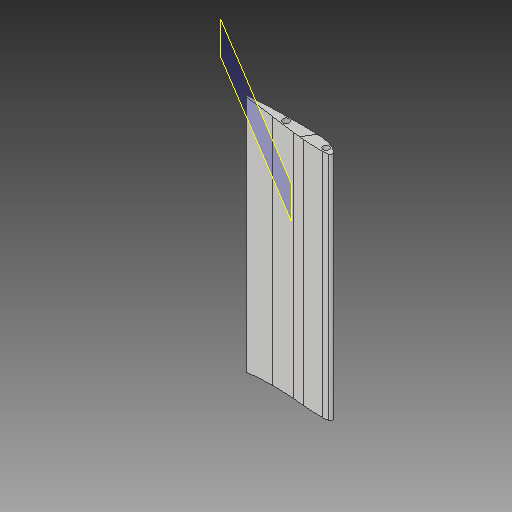
# Autodesk Inventor part: newsubflap_top
Saved by Autodesk Inventor 2018.3 (Build 223284000, 284)
## iProperties
Created: 2018-06-11
Part Number: newsubflap_top
Material: 一般
Document SubType Name: Modeling
Designer: ku_sk
Density: 1 g/cm^3
Appearance: 既定
Author: ku_sk
Autodesk Inventor part; units mm, degrees
ref_plane "YZ Plane" through (0, 0, 0) normal (1, 0, 0) x (0, 1, 0)
ref_plane "XZ Plane" through (0, 0, 0) normal (0, 1, 0) x (-1, 0, 0)
ref_plane "XY Plane" through (0, 0, 0) normal (0, 0, 1) x (1, 0, 0)
sketch "スケッチ1" plane through (0, 0, 0) normal (0, 1, 0) x (-1, 0, 0)
  circle A0 centre (56.6667, -3.3333) radius 2 projected
  circle A1 centre (6.6667, -1.3333) radius 2 projected
  arc A2 (27.618, -9.313) -> (80.2911, 0.2239) centre (24.5838, 157.671) ccw projected
  arc A3 (20.5062, -9.2317) -> (27.618, -9.313) centre (25.435, 110.8283) ccw projected
  arc A4 (7.5483, -6.9284) -> (20.5062, -9.2317) centre (22.5133, 39.66) ccw projected
  arc A5 (0.14, -3.2897) -> (7.5483, -6.9284) centre (16.2383, 20.125) ccw projected
  arc A6 (-1.8521, -1.3552) -> (0.14, -3.2897) centre (4.8333, 3.5367) ccw projected
  arc A7 (-0.4054, 2.2589) -> (-1.8521, -1.3552) centre (0, 0) ccw projected
  arc A8 (5.081, 2.7563) -> (-0.4054, 2.2589) centre (5.1833, -28.88) ccw projected
  arc A9 (23.6457, 1.9287) -> (5.081, 2.7563) centre (5.71, -191.7767) ccw projected
  arc A10 (23.6457, 1.9287) -> (35.0642, 0.89) centre (351.2983, 3540.5833) ccw projected
  arc A11 (35.0642, 0.89) -> (56.4197, -0.0064) centre (55.24, 226.7233) ccw projected
  arc A12 (56.4197, -0.0064) -> (79.9865, 1.514) centre (55.3817, 199.4967) ccw projected
  arc A13 (80.2911, 0.2239) -> (79.9865, 1.514) centre (80.0687, 0.8524) ccw projected
extrude "押し出し1" add sketch "スケッチ1" along normal mid plane 250 contours A0 | A1 | A3 A4 A5 A6 A7 A8 A9 A10 A11 A12 A13 A2
sketch "スケッチ2" plane through (0, -125, 0) normal (0, -1, 0) x (1, 0, 0)
  circle A0 centre (-6, -2) radius 3
  circle A1 centre (-47, -4) radius 3
  point P0 (0, 0)
  dimension "d3" = 6
  dimension "d4" = 6
  dimension "d5" = 6
  dimension "d6" = 2
  dimension "d7" = 4
  dimension "d8" = 47
  constraints: 2 centre point
  measures "d3" diameter of A0
  measures "d4" diameter of A1
  measures "d5" horizontal distance of A0.centre point (0, 0)
  measures "d6" vertical distance of point (0, 0) A0.centre
  measures "d7" vertical distance of point (0, 0) A1.centre
  measures "d8" horizontal distance of point (0, 0) A1.centre
extrude "押し出し2" cut sketch "スケッチ2" against normal through all
ref_plane "作業平面1" through (-121.5758, 135, -17.9326) normal (0.5160429, 0, -0.8565628) x (0.8565628, 0, 0.5160429)
sketch "スケッチ4" plane through (-121.5758, 135, -17.9326) normal (0.5160429, 0, -0.8565628) x (0.8565628, 0, 0.5160429)
  arc A0 (90, 35) -> (0, 0) centre (90, -98.2143) ccw projected
  line L0 (183.3333, 35) -> (90, 35) projected
  line L1 (183.3333, 35) -> (183.3333, 0)
  line L2 (183.3333, 0) -> (0, 0)
  point P0 (113.3913, 135)
  constraints: 4 end point, 1 perpendicular, 1 vertical
extrude "押し出し4" cut sketch "スケッチ4" along normal through all
equation "\"d4\" = d3"
